Autodesk Inventor part; units mm, degrees
(part 4 of 7)
  arc A284 (154.8425, 86.3766) -> (155.0844, 86.0651) centre (160.0222, 90.1488) ccw projected
  arc A285 (154.6673, 86.6328) -> (154.8425, 86.3766) centre (159.1041, 89.4801) ccw projected
  arc A286 (154.3066, 86.5156) -> (154.6673, 86.6328) centre (148.5, 105) ccw projected
  arc A287 (154.3154, 86.2053) -> (154.3066, 86.5156) centre (149.0434, 86.2112) ccw projected
  arc A288 (154.3028, 85.8111) -> (154.3154, 86.2053) centre (147.9076, 86.2125) ccw projected
  arc A289 (154.2565, 85.3248) -> (154.3028, 85.8111) centre (146.7304, 86.2864) ccw projected
  arc A290 (153.872, 85.2164) -> (154.2565, 85.3248) centre (148.5, 105) ccw projected
  arc A291 (153.5785, 85.6068) -> (153.872, 85.2164) centre (159.7867, 89.9687) ccw projected
  arc A292 (153.3618, 85.9364) -> (153.5785, 85.6068) centre (158.8215, 89.2905) ccw projected
  arc A293 (153.2072, 86.2055) -> (153.3618, 85.9364) centre (157.8537, 88.696) ccw projected
  arc A294 (152.8384, 86.117) -> (153.2072, 86.2055) centre (148.5, 105) ccw projected
  arc A295 (152.8228, 85.807) -> (152.8384, 86.117) centre (147.5676, 86.2265) ccw projected
  arc A296 (152.7793, 85.415) -> (152.8228, 85.807) centre (146.4354, 86.3169) ccw projected
  arc A297 (152.6951, 84.9338) -> (152.7793, 85.415) centre (145.2676, 86.483) ccw projected
  arc A298 (152.3033, 84.8559) -> (152.6951, 84.9338) centre (148.5, 105) ccw projected
  arc A299 (152.0413, 85.2682) -> (152.3033, 84.8559) centre (158.5726, 89.1295) ccw projected
  arc A300 (151.8511, 85.6137) -> (152.0413, 85.2682) centre (157.5571, 88.5292) ccw projected
  arc A301 (151.7181, 85.8941) -> (151.8511, 85.6137) centre (156.5457, 88.0124) ccw projected
  arc A302 (151.3435, 85.8348) -> (151.7181, 85.8941) centre (148.5, 105) ccw projected
  arc A303 (151.3036, 85.527) -> (151.3435, 85.8348) centre (146.0975, 86.3575) ccw projected
  arc A304 (151.2295, 85.1396) -> (151.3036, 85.527) centre (144.9759, 86.5365) ccw projected
  arc A305 (151.1078, 84.6665) -> (151.2295, 85.1396) centre (143.8247, 86.7936) ccw projected
  arc A306 (150.7111, 84.6196) -> (151.1078, 84.6665) centre (148.5, 105) ccw projected
  arc A307 (150.4822, 85.0511) -> (150.7111, 84.6196) centre (157.2963, 88.3881) ccw projected
  arc A308 (150.3197, 85.4105) -> (150.4822, 85.0511) centre (156.2369, 87.8693) ccw projected
  arc A309 (150.2091, 85.7005) -> (150.3197, 85.4105) centre (155.1881, 87.4335) ccw projected
  arc A310 (149.831, 85.6708) -> (150.2091, 85.7005) centre (148.5, 105) ccw projected
  arc A311 (149.7671, 85.367) -> (149.831, 85.6708) centre (144.6423, 86.6035) ccw projected
  arc A312 (149.6629, 84.9867) -> (149.7671, 85.367) centre (143.5382, 86.8699) ccw projected
  arc A313 (149.5044, 84.5246) -> (149.6629, 84.9867) centre (142.4106, 87.2166) ccw projected
  arc A314 (149.1052, 84.5089) -> (149.5044, 84.5246) centre (148.5, 105) ccw projected
  arc A315 (148.9109, 84.9571) -> (149.1052, 84.5089) centre (155.9658, 87.7492) ccw projected
  arc A316 (148.7771, 85.3281) -> (148.9109, 84.9571) centre (154.869, 87.3151) ccw projected
  arc A317 (148.6896, 85.6259) -> (148.7771, 85.3281) centre (153.7892, 86.9629) ccw projected
  arc A318 (148.3104, 85.6259) -> (148.6896, 85.6259) centre (148.5, 105) ccw projected
  arc A319 (148.2229, 85.3281) -> (148.3104, 85.6259) centre (143.2108, 86.9629) ccw projected
  arc A320 (148.0891, 84.9571) -> (148.2229, 85.3281) centre (142.131, 87.3151) ccw projected
  arc A321 (147.8948, 84.5089) -> (148.0891, 84.9571) centre (141.0342, 87.7492) ccw projected
  arc A322 (147.4956, 84.5246) -> (147.8948, 84.5089) centre (148.5, 105) ccw projected
  arc A323 (147.3371, 84.9867) -> (147.4956, 84.5246) centre (154.5894, 87.2166) ccw projected
  arc A324 (147.2329, 85.367) -> (147.3371, 84.9867) centre (153.4618, 86.8699) ccw projected
  arc A325 (147.169, 85.6708) -> (147.2329, 85.367) centre (152.3577, 86.6035) ccw projected
  arc A326 (146.7909, 85.7005) -> (147.169, 85.6708) centre (148.5, 105) ccw projected
  arc A327 (146.6803, 85.4105) -> (146.7909, 85.7005) centre (141.8119, 87.4335) ccw projected
  arc A328 (146.5178, 85.0511) -> (146.6803, 85.4105) centre (140.7631, 87.8693) ccw projected
  arc A329 (146.2889, 84.6196) -> (146.5178, 85.0511) centre (139.7037, 88.3881) ccw projected
  arc A330 (145.8922, 84.6665) -> (146.2889, 84.6196) centre (148.5, 105) ccw projected
  arc A331 (145.7705, 85.1396) -> (145.8922, 84.6665) centre (153.1753, 86.7936) ccw projected
  arc A332 (145.6964, 85.527) -> (145.7705, 85.1396) centre (152.0241, 86.5365) ccw projected
  arc A333 (145.6565, 85.8348) -> (145.6964, 85.527) centre (150.9025, 86.3575) ccw projected
  arc A334 (145.2819, 85.8941) -> (145.6565, 85.8348) centre (148.5, 105) ccw projected
  arc A335 (145.1489, 85.6137) -> (145.2819, 85.8941) centre (140.4543, 88.0124) ccw projected
  arc A336 (144.9587, 85.2682) -> (145.1489, 85.6137) centre (139.4429, 88.5292) ccw projected
  arc A337 (144.6967, 84.8559) -> (144.9587, 85.2682) centre (138.4274, 89.1295) ccw projected
  arc A338 (144.3049, 84.9338) -> (144.6967, 84.8559) centre (148.5, 105) ccw projected
  arc A339 (144.2207, 85.415) -> (144.3049, 84.9338) centre (151.7324, 86.483) ccw projected
  arc A340 (144.1772, 85.807) -> (144.2207, 85.415) centre (150.5646, 86.3169) ccw projected
  arc A341 (144.1616, 86.117) -> (144.1772, 85.807) centre (149.4324, 86.2265) ccw projected
  arc A342 (143.7928, 86.2055) -> (144.1616, 86.117) centre (148.5, 105) ccw projected
  arc A343 (143.6382, 85.9364) -> (143.7928, 86.2055) centre (139.1463, 88.696) ccw projected
  arc A344 (143.4215, 85.6068) -> (143.6382, 85.9364) centre (138.1785, 89.2905) ccw projected
  arc A345 (143.128, 85.2164) -> (143.4215, 85.6068) centre (137.2133, 89.9687) ccw projected
  arc A346 (142.7435, 85.3248) -> (143.128, 85.2164) centre (148.5, 105) ccw projected
  arc A347 (142.6972, 85.8111) -> (142.7435, 85.3248) centre (150.2696, 86.2864) ccw projected
  arc A348 (142.6846, 86.2053) -> (142.6972, 85.8111) centre (149.0924, 86.2125) ccw projected
  arc A349 (142.6934, 86.5156) -> (142.6846, 86.2053) centre (147.9566, 86.2112) ccw projected
  arc A350 (142.3327, 86.6328) -> (142.6934, 86.5156) centre (148.5, 105) ccw projected
  arc A351 (142.1575, 86.3766) -> (142.3327, 86.6328) centre (137.8959, 89.4801) ccw projected
  arc A352 (141.9156, 86.0651) -> (142.1575, 86.3766) centre (136.9778, 90.1488) ccw projected
  arc A353 (141.5923, 85.6989) -> (141.9156, 86.0651) centre (136.0688, 90.9006) ccw projected
  arc A354 (141.2175, 85.8371) -> (141.5923, 85.6989) centre (148.5, 105) ccw projected
  arc A355 (141.2096, 86.3255) -> (141.2175, 85.8371) centre (148.7959, 86.2053) ccw projected
  arc A356 (141.228, 86.7195) -> (141.2096, 86.3255) centre (147.6165, 86.224) ccw projected
  arc A357 (141.2611, 87.0281) -> (141.228, 86.7195) centre (146.4841, 86.3118) ccw projected
  arc A358 (140.9107, 87.1733) -> (141.2611, 87.0281) centre (148.5, 105) ccw projected
  arc A359 (140.7158, 86.9316) -> (140.9107, 87.1733) centre (136.7109, 90.36) ccw projected
  arc A360 (140.4503, 86.64) -> (140.7158, 86.9316) centre (135.8481, 91.0986) ccw projected
  arc A361 (140.0993, 86.3003) -> (140.4503, 86.64) centre (135.0009, 91.9194) ccw projected
  arc A362 (139.7365, 86.4676) -> (140.0993, 86.3003) centre (148.5, 105) ccw projected
  arc A363 (139.7669, 86.9551) -> (139.7365, 86.4676) centre (147.3204, 86.24) ccw projected
  arc A364 (139.8161, 87.3464) -> (139.7669, 86.9551) centre (146.1461, 86.3512) ccw projected
  arc A365 (139.8733, 87.6515) -> (139.8161, 87.3464) centre (145.024, 86.5276) ccw projected
  arc A366 (139.5354, 87.8237) -> (139.8733, 87.6515) centre (148.5, 105) ccw projected
  arc A367 (139.3222, 87.5981) -> (139.5354, 87.8237) centre (135.5986, 91.3301) ccw projected
  arc A368 (139.0346, 87.3282) -> (139.3222, 87.5981) centre (134.7964, 92.1341) ccw projected
  arc A369 (138.658, 87.0171) -> (139.0346, 87.3282) centre (134.0162, 93.0188) ccw projected
  arc A370 (138.3095, 87.2123) -> (138.658, 87.0171) centre (148.5, 105) ccw projected
  arc A371 (138.378, 87.6959) -> (138.3095, 87.2123) centre (145.8522, 86.3904) ccw projected
  arc A372 (138.4578, 88.0822) -> (138.378, 87.6959) centre (144.6901, 86.5933) ccw projected
  arc A373 (138.5388, 88.3818) -> (138.4578, 88.0822) centre (143.5854, 86.8572) ccw projected
  arc A374 (138.2154, 88.58) -> (138.5388, 88.3818) centre (148.5, 105) ccw projected
  arc A375 (137.9852, 88.3718) -> (138.2154, 88.58) centre (134.5659, 92.3844) ccw projected
  arc A376 (137.6773, 88.1253) -> (137.9852, 88.3718) centre (133.8292, 93.2489) ccw projected
  arc A377 (137.2774, 87.8447) -> (137.6773, 88.1253) centre (133.1208, 94.1922) ccw projected
  arc A378 (136.9453, 88.0666) -> (137.2774, 87.8447) centre (148.5, 105) ccw projected
  arc A379 (137.0515, 88.5434) -> (136.9453, 88.0666) centre (144.4002, 86.6555) ccw projected
  arc A380 (137.1614, 88.9222) -> (137.0515, 88.5434) centre (143.2577, 86.949) ccw projected
  arc A381 (137.2656, 89.2146) -> (137.1614, 88.9222) centre (142.1771, 87.2988) ccw projected
  arc A382 (136.9588, 89.4375) -> (137.2656, 89.2146) centre (148.5, 105) ccw projected
  arc A383 (136.7129, 89.248) -> (136.9588, 89.4375) centre (133.619, 93.5166) ccw projected
  arc A384 (136.3866, 89.0265) -> (136.7129, 89.248) centre (132.9524, 94.4362) ccw projected
  arc A385 (135.966, 88.7781) -> (136.3866, 89.0265) centre (132.3202, 95.4321) ccw projected
  arc A386 (135.6523, 89.0254) -> (135.966, 88.7781) centre (148.5, 105) ccw projected
  arc A387 (135.7957, 89.4924) -> (135.6523, 89.0254) centre (142.9736, 87.0337) ccw projected
  arc A388 (135.9349, 89.8614) -> (135.7957, 89.4924) centre (141.8576, 87.4159) ccw projected
  arc A389 (136.0617, 90.1447) -> (135.9349, 89.8614) centre (140.8078, 87.8494) ccw projected
  arc A390 (135.7734, 90.391) -> (136.0617, 90.1447) centre (148.5, 105) ccw projected
  arc A391 (135.5134, 90.2214) -> (135.7734, 90.391) centre (132.7639, 94.7195) ccw projected
  arc A392 (135.1707, 90.0261) -> (135.5134, 90.2214) centre (132.1715, 95.6886) ccw projected
  arc A393 (134.7319, 89.8115) -> (135.1707, 90.0261) centre (131.6194, 96.7311) ccw projected
  arc A394 (134.4386, 90.0827) -> (134.7319, 89.8115) centre (148.5, 105) ccw projected
  arc A395 (134.6181, 90.537) -> (134.4386, 90.0827) centre (141.581, 87.5227) ccw projected
  arc A396 (134.7859, 90.8939) -> (134.6181, 90.537) centre (140.4985, 87.9913) ccw projected
  arc A397 (134.9345, 91.1664) -> (134.7859, 90.8939) centre (139.4859, 88.5058) ccw projected
  arc A398 (134.6664, 91.4345) -> (134.9345, 91.1664) centre (148.5, 105) ccw projected
  arc A399 (134.3939, 91.2859) -> (134.6664, 91.4345) centre (132.0058, 95.9859) ccw projected
  arc A400 (134.037, 91.1181) -> (134.3939, 91.2859) centre (131.4913, 96.9985) ccw projected
  arc A401 (133.5827, 90.9386) -> (134.037, 91.1181) centre (131.0227, 98.081) ccw projected
  arc A402 (133.3115, 91.2319) -> (133.5827, 90.9386) centre (148.5, 105) ccw projected
  arc A403 (133.5261, 91.6707) -> (133.3115, 91.2319) centre (140.2311, 88.1194) ccw projected
  arc A404 (133.7214, 92.0134) -> (133.5261, 91.6707) centre (139.1886, 88.6715) ccw projected
  arc A405 (133.891, 92.2734) -> (133.7214, 92.0134) centre (138.2195, 89.2639) ccw projected
  arc A406 (133.6447, 92.5617) -> (133.891, 92.2734) centre (148.5, 105) ccw projected
  arc A407 (133.3614, 92.4349) -> (133.6447, 92.5617) centre (131.3494, 97.3078) ccw projected
  arc A408 (132.9924, 92.2957) -> (133.3614, 92.4349) centre (130.9159, 98.3576) ccw projected
  arc A409 (132.5254, 92.1523) -> (132.9924, 92.2957) centre (130.5337, 99.4736) ccw projected
  arc A410 (132.2781, 92.466) -> (132.5254, 92.1523) centre (148.5, 105) ccw projected
  arc A411 (132.5265, 92.8866) -> (132.2781, 92.466) centre (138.9321, 88.8202) ccw projected
  arc A412 (132.748, 93.2129) -> (132.5265, 92.8866) centre (137.9362, 89.4524) ccw projected
  arc A413 (132.9375, 93.4588) -> (132.748, 93.2129) centre (137.0166, 90.119) ccw projected
  arc A414 (132.7146, 93.7656) -> (132.9375, 93.4588) centre (148.5, 105) ccw projected
  arc A415 (132.4222, 93.6614) -> (132.7146, 93.7656) centre (130.7988, 98.6771) ccw projected
  arc A416 (132.0434, 93.5515) -> (132.4222, 93.6614) centre (130.449, 99.7577) ccw projected
  arc A417 (131.5666, 93.4453) -> (132.0434, 93.5515) centre (130.1555, 100.9002) ccw projected
  arc A418 (131.3447, 93.7774) -> (131.5666, 93.4453) centre (148.5, 105) ccw projected
  arc A419 (131.6253, 94.1773) -> (131.3447, 93.7774) centre (137.6922, 89.6208) ccw projected
  arc A420 (131.8718, 94.4852) -> (131.6253, 94.1773) centre (136.7489, 90.3292) ccw projected
  arc A421 (132.08, 94.7154) -> (131.8718, 94.4852) centre (135.8844, 91.0659) ccw projected
  arc A422 (131.8818, 95.0388) -> (132.08, 94.7154) centre (148.5, 105) ccw projected
  arc A423 (131.5822, 94.9578) -> (131.8818, 95.0388) centre (130.3572, 100.0854) ccw projected
  arc A424 (131.1959, 94.878) -> (131.5822, 94.9578) centre (130.0933, 101.1901) ccw projected
  arc A425 (130.7123, 94.8095) -> (131.1959, 94.878) centre (129.8904, 102.3522) ccw projected
  arc A426 (130.5171, 95.158) -> (130.7123, 94.8095) centre (148.5, 105) ccw projected
  arc A427 (130.8282, 95.5346) -> (130.5171, 95.158) centre (136.5188, 90.5162) ccw projected
  arc A428 (131.0981, 95.8222) -> (130.8282, 95.5346) centre (135.6341, 91.2964) ccw projected
  arc A429 (131.3237, 96.0354) -> (131.0981, 95.8222) centre (134.8301, 92.0986) ccw projected
  arc A430 (131.1515, 96.3733) -> (131.3237, 96.0354) centre (148.5, 105) ccw projected
  arc A431 (130.8464, 96.3161) -> (131.1515, 96.3733) centre (130.0276, 101.524) ccw projected
  arc A432 (130.4551, 96.2669) -> (130.8464, 96.3161) centre (129.8512, 102.6461) ccw projected
  arc A433 (129.9676, 96.2365) -> (130.4551, 96.2669) centre (129.74, 103.8204) ccw projected
  arc A434 (129.8003, 96.5993) -> (129.9676, 96.2365) centre (148.5, 105) ccw projected
  arc A435 (130.14, 96.9503) -> (129.8003, 96.5993) centre (135.4194, 91.5009) ccw projected
  arc A436 (130.4316, 97.2158) -> (130.14, 96.9503) centre (134.5986, 92.3481) ccw projected
  arc A437 (130.6733, 97.4107) -> (130.4316, 97.2158) centre (133.86, 93.2109) ccw projected
  arc A438 (130.5281, 97.7611) -> (130.6733, 97.4107) centre (148.5, 105) ccw projected
  arc A439 (130.2195, 97.728) -> (130.5281, 97.7611) centre (129.8118, 102.9841) ccw projected
  arc A440 (129.8255, 97.7096) -> (130.2195, 97.728) centre (129.724, 104.1165) ccw projected
  arc A441 (129.3371, 97.7175) -> (129.8255, 97.7096) centre (129.7053, 105.2959) ccw projected
  arc A442 (129.1989, 98.0923) -> (129.3371, 97.7175) centre (148.5, 105) ccw projected
  arc A443 (129.5651, 98.4156) -> (129.1989, 98.0923) centre (134.4006, 92.5688) ccw projected
  arc A444 (129.8766, 98.6575) -> (129.5651, 98.4156) centre (133.6488, 93.4778) ccw projected
  arc A445 (130.1328, 98.8327) -> (129.8766, 98.6575) centre (132.9801, 94.3959) ccw projected
  arc A446 (130.0156, 99.1934) -> (130.1328, 98.8327) centre (148.5, 105) ccw projected
  arc A447 (129.7053, 99.1846) -> (130.0156, 99.1934) centre (129.7112, 104.4566) ccw projected
  arc A448 (129.3111, 99.1972) -> (129.7053, 99.1846) centre (129.7125, 105.5924) ccw projected
  arc A449 (128.8248, 99.2435) -> (129.3111, 99.1972) centre (129.7864, 106.7696) ccw projected
  arc A450 (128.7164, 99.628) -> (128.8248, 99.2435) centre (148.5, 105) ccw projected
  arc A451 (129.1068, 99.9215) -> (128.7164, 99.628) centre (133.4687, 93.7133) ccw projected
  arc A452 (129.4364, 100.1382) -> (129.1068, 99.9215) centre (132.7905, 94.6785) ccw projected
  arc A453 (129.7055, 100.2928) -> (129.4364, 100.1382) centre (132.196, 95.6463) ccw projected
  arc A454 (129.617, 100.6616) -> (129.7055, 100.2928) centre (148.5, 105) ccw projected
  arc A455 (129.307, 100.6772) -> (129.617, 100.6616) centre (129.7265, 105.9324) ccw projected
  arc A456 (128.915, 100.7207) -> (129.307, 100.6772) centre (129.8169, 107.0646) ccw projected
  arc A457 (128.4338, 100.8049) -> (128.915, 100.7207) centre (129.983, 108.2324) ccw projected
  arc A458 (128.3559, 101.1967) -> (128.4338, 100.8049) centre (148.5, 105) ccw projected
  arc A459 (128.7682, 101.4587) -> (128.3559, 101.1967) centre (132.6295, 94.9274) ccw projected
  arc A460 (129.1137, 101.6489) -> (128.7682, 101.4587) centre (132.0292, 95.9429) ccw projected
  arc A461 (129.3941, 101.7819) -> (129.1137, 101.6489) centre (131.5124, 96.9543) ccw projected
  arc A462 (129.3348, 102.1565) -> (129.3941, 101.7819) centre (148.5, 105) ccw projected
  arc A463 (129.027, 102.1964) -> (129.3348, 102.1565) centre (129.8575, 107.4025) ccw projected
  arc A464 (128.6396, 102.2705) -> (129.027, 102.1964) centre (130.0365, 108.5241) ccw projected
  arc A465 (128.1665, 102.3922) -> (128.6396, 102.2705) centre (130.2936, 109.6753) ccw projected
  arc A466 (128.1196, 102.7889) -> (128.1665, 102.3922) centre (148.5, 105) ccw projected
  arc A467 (128.5511, 103.0178) -> (128.1196, 102.7889) centre (131.8881, 96.2037) ccw projected
  arc A468 (128.9105, 103.1803) -> (128.5511, 103.0178) centre (131.3693, 97.2631) ccw projected
  arc A469 (129.2005, 103.2909) -> (128.9105, 103.1803) centre (130.9335, 98.3119) ccw projected
  arc A470 (129.1708, 103.669) -> (129.2005, 103.2909) centre (148.5, 105) ccw projected
  arc A471 (128.867, 103.7329) -> (129.1708, 103.669) centre (130.1035, 108.8577) ccw projected
  arc A472 (128.4867, 103.8371) -> (128.867, 103.7329) centre (130.3699, 109.9618) ccw projected
  arc A473 (128.0246, 103.9956) -> (128.4867, 103.8371) centre (130.7166, 111.0894) ccw projected
  arc A474 (128.0089, 104.3948) -> (128.0246, 103.9956) centre (148.5, 105) ccw projected
  arc A475 (128.4571, 104.5891) -> (128.0089, 104.3948) centre (131.2492, 97.5342) ccw projected
  arc A476 (128.8281, 104.7229) -> (128.4571, 104.5891) centre (130.8151, 98.631) ccw projected
  arc A477 (129.1259, 104.8104) -> (128.8281, 104.7229) centre (130.4629, 99.7108) ccw projected
  arc A478 (129.1259, 105.1896) -> (129.1259, 104.8104) centre (148.5, 105) ccw projected
  arc A479 (128.8281, 105.2771) -> (129.1259, 105.1896) centre (130.4629, 110.2892) ccw projected
  arc A480 (128.4571, 105.4109) -> (128.8281, 105.2771) centre (130.8151, 111.369) ccw projected
  arc A481 (128.0089, 105.6052) -> (128.4571, 105.4109) centre (131.2492, 112.4658) ccw projected
  arc A482 (128.0246, 106.0044) -> (128.0089, 105.6052) centre (148.5, 105) ccw projected
  arc A483 (128.4867, 106.1629) -> (128.0246, 106.0044) centre (130.7166, 98.9106) ccw projected
  arc A484 (128.867, 106.2671) -> (128.4867, 106.1629) centre (130.3699, 100.0382) ccw projected
  arc A485 (129.1708, 106.331) -> (128.867, 106.2671) centre (130.1035, 101.1423) ccw projected
  arc A486 (129.2005, 106.7091) -> (129.1708, 106.331) centre (148.5, 105) ccw projected
  arc A487 (128.9105, 106.8197) -> (129.2005, 106.7091) centre (130.9335, 111.6881) ccw projected
  arc A488 (128.5511, 106.9822) -> (128.9105, 106.8197) centre (131.3693, 112.7369) ccw projected
  arc A489 (128.1196, 107.2111) -> (128.5511, 106.9822) centre (131.8881, 113.7963) ccw projected
  arc A490 (128.1665, 107.6078) -> (128.1196, 107.2111) centre (148.5, 105) ccw projected
  arc A491 (128.6396, 107.7295) -> (128.1665, 107.6078) centre (130.2936, 100.3247) ccw projected
  arc A492 (129.027, 107.8036) -> (128.6396, 107.7295) centre (130.0365, 101.4759) ccw projected
  arc A493 (129.3348, 107.8435) -> (129.027, 107.8036) centre (129.8575, 102.5975) ccw projected
  arc A494 (129.3941, 108.2181) -> (129.3348, 107.8435) centre (148.5, 105) ccw projected
  arc A495 (129.1137, 108.3511) -> (129.3941, 108.2181) centre (131.5124, 113.0457) ccw projected
  arc A496 (128.7682, 108.5413) -> (129.1137, 108.3511) centre (132.0292, 114.0571) ccw projected
  arc A497 (128.3559, 108.8033) -> (128.7682, 108.5413) centre (132.6295, 115.0726) ccw projected
  arc A498 (128.4338, 109.1951) -> (128.3559, 108.8033) centre (148.5, 105) ccw projected
  arc A499 (128.915, 109.2793) -> (128.4338, 109.1951) centre (129.983, 101.7676) ccw projected
  arc A500 (129.307, 109.3228) -> (128.915, 109.2793) centre (129.8169, 102.9354) ccw projected
  arc A501 (129.617, 109.3384) -> (129.307, 109.3228) centre (129.7265, 104.0676) ccw projected
  arc A502 (129.7055, 109.7072) -> (129.617, 109.3384) centre (148.5, 105) ccw projected
  arc A503 (129.4364, 109.8618) -> (129.7055, 109.7072) centre (132.196, 114.3537) ccw projected
  arc A504 (129.1068, 110.0785) -> (129.4364, 109.8618) centre (132.7905, 115.3215) ccw projected
  arc A505 (128.7164, 110.372) -> (129.1068, 110.0785) centre (133.4687, 116.2867) ccw projected
  arc A506 (128.8248, 110.7565) -> (128.7164, 110.372) centre (148.5, 105) ccw projected
  arc A507 (129.3111, 110.8028) -> (128.8248, 110.7565) centre (129.7864, 103.2304) ccw projected
  arc A508 (129.7053, 110.8154) -> (129.3111, 110.8028) centre (129.7125, 104.4076) ccw projected
  arc A509 (130.0156, 110.8066) -> (129.7053, 110.8154) centre (129.7112, 105.5434) ccw projected
  arc A510 (130.1328, 111.1673) -> (130.0156, 110.8066) centre (148.5, 105) ccw projected
  arc A511 (129.8766, 111.3425) -> (130.1328, 111.1673) centre (132.9801, 115.6041) ccw projected
  arc A512 (129.5651, 111.5844) -> (129.8766, 111.3425) centre (133.6488, 116.5222) ccw projected
  arc A513 (129.1989, 111.9077) -> (129.5651, 111.5844) centre (134.4006, 117.4312) ccw projected
  arc A514 (129.3371, 112.2825) -> (129.1989, 111.9077) centre (148.5, 105) ccw projected
  arc A515 (129.8255, 112.2904) -> (129.3371, 112.2825) centre (129.7053, 104.7041) ccw projected
  arc A516 (130.2195, 112.272) -> (129.8255, 112.2904) centre (129.724, 105.8835) ccw projected
  arc A517 (130.5281, 112.2389) -> (130.2195, 112.272) centre (129.8118, 107.0159) ccw projected
  arc A518 (130.6733, 112.5893) -> (130.5281, 112.2389) centre (148.5, 105) ccw projected
  arc A519 (130.4316, 112.7842) -> (130.6733, 112.5893) centre (133.86, 116.7891) ccw projected
  arc A520 (130.14, 113.0497) -> (130.4316, 112.7842) centre (134.5986, 117.6519) ccw projected
  arc A521 (129.8003, 113.4007) -> (130.14, 113.0497) centre (135.4194, 118.4991) ccw projected
  arc A522 (129.9676, 113.7635) -> (129.8003, 113.4007) centre (148.5, 105) ccw projected
  arc A523 (130.4551, 113.7331) -> (129.9676, 113.7635) centre (129.74, 106.1796) ccw projected
  arc A524 (130.8464, 113.6839) -> (130.4551, 113.7331) centre (129.8512, 107.3539) ccw projected
  arc A525 (131.1515, 113.6267) -> (130.8464, 113.6839) centre (130.0276, 108.476) ccw projected
  arc A526 (131.3237, 113.9646) -> (131.1515, 113.6267) centre (148.5, 105) ccw projected
  arc A527 (131.0981, 114.1778) -> (131.3237, 113.9646) centre (134.8301, 117.9014) ccw projected
  arc A528 (130.8282, 114.4654) -> (131.0981, 114.1778) centre (135.6341, 118.7036) ccw projected
  arc A529 (130.5171, 114.842) -> (130.8282, 114.4654) centre (136.5188, 119.4838) ccw projected
  arc A530 (130.7123, 115.1905) -> (130.5171, 114.842) centre (148.5, 105) ccw projected
  arc A531 (131.1959, 115.122) -> (130.7123, 115.1905) centre (129.8904, 107.6478) ccw projected
  arc A532 (131.5822, 115.0422) -> (131.1959, 115.122) centre (130.0933, 108.8099) ccw projected
  arc A533 (131.8818, 114.9612) -> (131.5822, 115.0422) centre (130.3572, 109.9146) ccw projected
  arc A534 (132.08, 115.2846) -> (131.8818, 114.9612) centre (148.5, 105) ccw projected
  arc A535 (131.8718, 115.5148) -> (132.08, 115.2846) centre (135.8844, 118.9341) ccw projected
  arc A536 (131.6253, 115.8227) -> (131.8718, 115.5148) centre (136.7489, 119.6708) ccw projected
  arc A537 (131.3447, 116.2226) -> (131.6253, 115.8227) centre (137.6922, 120.3792) ccw projected
  arc A538 (131.5666, 116.5547) -> (131.3447, 116.2226) centre (148.5, 105) ccw projected
  arc A539 (132.0434, 116.4485) -> (131.5666, 116.5547) centre (130.1555, 109.0998) ccw projected
  arc A540 (132.4222, 116.3386) -> (132.0434, 116.4485) centre (130.449, 110.2423) ccw projected
  arc A541 (132.7146, 116.2344) -> (132.4222, 116.3386) centre (130.7988, 111.3229) ccw projected
  arc A542 (132.9375, 116.5412) -> (132.7146, 116.2344) centre (148.5, 105) ccw projected
  arc A543 (132.748, 116.7871) -> (132.9375, 116.5412) centre (137.0166, 119.881) ccw projected
  arc A544 (132.5265, 117.1134) -> (132.748, 116.7871) centre (137.9362, 120.5476) ccw projected
  arc A545 (132.2781, 117.534) -> (132.5265, 117.1134) centre (138.9321, 121.1798) ccw projected
  arc A546 (132.5254, 117.8477) -> (132.2781, 117.534) centre (148.5, 105) ccw projected
  arc A547 (132.9924, 117.7043) -> (132.5254, 117.8477) centre (130.5337, 110.5264) ccw projected
  arc A548 (133.3614, 117.5651) -> (132.9924, 117.7043) centre (130.9159, 111.6424) ccw projected
  arc A549 (133.6447, 117.4383) -> (133.3614, 117.5651) centre (131.3494, 112.6922) ccw projected
  arc A550 (133.891, 117.7266) -> (133.6447, 117.4383) centre (148.5, 105) ccw projected
  arc A551 (133.7214, 117.9866) -> (133.891, 117.7266) centre (138.2195, 120.7361) ccw projected
  arc A552 (133.5261, 118.3293) -> (133.7214, 117.9866) centre (139.1886, 121.3285) ccw projected
  arc A553 (133.3115, 118.7681) -> (133.5261, 118.3293) centre (140.2311, 121.8806) ccw projected
  arc A554 (133.5827, 119.0614) -> (133.3115, 118.7681) centre (148.5, 105) ccw projected
  arc A555 (134.037, 118.8819) -> (133.5827, 119.0614) centre (131.0227, 111.919) ccw projected
  arc A556 (134.3939, 118.7141) -> (134.037, 118.8819) centre (131.4913, 113.0015) ccw projected
  arc A557 (134.6664, 118.5655) -> (134.3939, 118.7141) centre (132.0058, 114.0141) ccw projected
  arc A558 (134.9345, 118.8336) -> (134.6664, 118.5655) centre (148.5, 105) ccw projected
  arc A559 (134.7859, 119.1061) -> (134.9345, 118.8336) centre (139.4859, 121.4942) ccw projected
  arc A560 (134.6181, 119.463) -> (134.7859, 119.1061) centre (140.4985, 122.0087) ccw projected
  arc A561 (134.4386, 119.9173) -> (134.6181, 119.463) centre (141.581, 122.4773) ccw projected
  arc A562 (134.7319, 120.1885) -> (134.4386, 119.9173) centre (148.5, 105) ccw projected
  arc A563 (135.1707, 119.9739) -> (134.7319, 120.1885) centre (131.6194, 113.2689) ccw projected
  arc A564 (135.5134, 119.7786) -> (135.1707, 119.9739) centre (132.1715, 114.3114) ccw projected
  arc A565 (135.7734, 119.609) -> (135.5134, 119.7786) centre (132.7639, 115.2805) ccw projected
  arc A566 (136.0617, 119.8553) -> (135.7734, 119.609) centre (148.5, 105) ccw projected
  arc A567 (135.9349, 120.1386) -> (136.0617, 119.8553) centre (140.8078, 122.1506) ccw projected
  arc A568 (135.7957, 120.5076) -> (135.9349, 120.1386) centre (141.8576, 122.5841) ccw projected
  arc A569 (135.6523, 120.9746) -> (135.7957, 120.5076) centre (142.9736, 122.9663) ccw projected
  arc A570 (135.966, 121.2219) -> (135.6523, 120.9746) centre (148.5, 105) ccw projected
  arc A571 (136.3866, 120.9735) -> (135.966, 121.2219) centre (132.3202, 114.5679) ccw projected
  arc A572 (136.7129, 120.752) -> (136.3866, 120.9735) centre (132.9524, 115.5638) ccw projected
  arc A573 (136.9588, 120.5625) -> (136.7129, 120.752) centre (133.619, 116.4834) ccw projected
  arc A574 (137.2656, 120.7854) -> (136.9588, 120.5625) centre (148.5, 105) ccw projected
  arc A575 (137.1614, 121.0778) -> (137.2656, 120.7854) centre (142.1771, 122.7012) ccw projected
  arc A576 (137.0515, 121.4566) -> (137.1614, 121.0778) centre (143.2577, 123.051) ccw projected
  arc A577 (136.9453, 121.9334) -> (137.0515, 121.4566) centre (144.4002, 123.3445) ccw projected
  arc A578 (137.2774, 122.1553) -> (136.9453, 121.9334) centre (148.5, 105) ccw projected
  arc A579 (137.6773, 121.8747) -> (137.2774, 122.1553) centre (133.1208, 115.8078) ccw projected
  arc A580 (137.9852, 121.6282) -> (137.6773, 121.8747) centre (133.8292, 116.7511) ccw projected
  arc A581 (138.2154, 121.42) -> (137.9852, 121.6282) centre (134.5659, 117.6156) ccw projected
  arc A582 (138.5388, 121.6182) -> (138.2154, 121.42) centre (148.5, 105) ccw projected
  arc A583 (138.4578, 121.9178) -> (138.5388, 121.6182) centre (143.5854, 123.1428) ccw projected
  arc A584 (138.378, 122.3041) -> (138.4578, 121.9178) centre (144.6901, 123.4067) ccw projected
  arc A585 (138.3095, 122.7877) -> (138.378, 122.3041) centre (145.8522, 123.6096) ccw projected
  arc A586 (138.658, 122.9829) -> (138.3095, 122.7877) centre (148.5, 105) ccw projected
  arc A587 (139.0346, 122.6718) -> (138.658, 122.9829) centre (134.0162, 116.9812) ccw projected
  arc A588 (139.3222, 122.4019) -> (139.0346, 122.6718) centre (134.7964, 117.8659) ccw projected
  arc A589 (139.5354, 122.1763) -> (139.3222, 122.4019) centre (135.5986, 118.6699) ccw projected
  arc A590 (139.8733, 122.3485) -> (139.5354, 122.1763) centre (148.5, 105) ccw projected
  arc A591 (139.8161, 122.6536) -> (139.8733, 122.3485) centre (145.024, 123.4724) ccw projected
  arc A592 (139.7669, 123.0449) -> (139.8161, 122.6536) centre (146.1461, 123.6488) ccw projected
  arc A593 (139.7365, 123.5324) -> (139.7669, 123.0449) centre (147.3204, 123.76) ccw projected
  arc A594 (140.0993, 123.6997) -> (139.7365, 123.5324) centre (148.5, 105) ccw projected
  arc A595 (140.4503, 123.36) -> (140.0993, 123.6997) centre (135.0009, 118.0806) ccw projected
  arc A596 (140.7158, 123.0684) -> (140.4503, 123.36) centre (135.8481, 118.9014) ccw projected
  arc A597 (140.9107, 122.8267) -> (140.7158, 123.0684) centre (136.7109, 119.64) ccw projected
  arc A598 (141.2611, 122.9719) -> (140.9107, 122.8267) centre (148.5, 105) ccw projected
  arc A599 (141.228, 123.2805) -> (141.2611, 122.9719) centre (146.4841, 123.6882) ccw projected
  arc A600 (141.2096, 123.6745) -> (141.228, 123.2805) centre (147.6165, 123.776) ccw projected
  arc A601 (141.2175, 124.1629) -> (141.2096, 123.6745) centre (148.7959, 123.7947) ccw projected
  arc A602 (141.5923, 124.3011) -> (141.2175, 124.1629) centre (148.5, 105) ccw projected
  arc A603 (141.9156, 123.9349) -> (141.5923, 124.3011) centre (136.0688, 119.0994) ccw projected
  arc A604 (142.1575, 123.6234) -> (141.9156, 123.9349) centre (136.9778, 119.8512) ccw projected
  arc A605 (142.3327, 123.3672) -> (142.1575, 123.6234) centre (137.8959, 120.5199) ccw projected
  arc A606 (142.6934, 123.4844) -> (142.3327, 123.3672) centre (148.5, 105) ccw projected
  arc A607 (142.6846, 123.7947) -> (142.6934, 123.4844) centre (147.9566, 123.7888) ccw projected
  arc A608 (142.6972, 124.1889) -> (142.6846, 123.7947) centre (149.0924, 123.7875) ccw projected
  arc A609 (142.7435, 124.6752) -> (142.6972, 124.1889) centre (150.2696, 123.7136) ccw projected
  arc A610 (143.128, 124.7836) -> (142.7435, 124.6752) centre (148.5, 105) ccw projected
  arc A611 (143.4215, 124.3932) -> (143.128, 124.7836) centre (137.2133, 120.0313) ccw projected
  arc A612 (143.6382, 124.0636) -> (143.4215, 124.3932) centre (138.1785, 120.7095) ccw projected
  arc A613 (143.7928, 123.7945) -> (143.6382, 124.0636) centre (139.1463, 121.304) ccw projected
  arc A614 (144.1616, 123.883) -> (143.7928, 123.7945) centre (148.5, 105) ccw projected
  arc A615 (144.1772, 124.193) -> (144.1616, 123.883) centre (149.4324, 123.7735) ccw projected
  arc A616 (144.2207, 124.585) -> (144.1772, 124.193) centre (150.5646, 123.6831) ccw projected
  arc A617 (144.3049, 125.0662) -> (144.2207, 124.585) centre (151.7324, 123.517) ccw projected
  arc A618 (144.6967, 125.1441) -> (144.3049, 125.0662) centre (148.5, 105) ccw projected
  arc A619 (144.9587, 124.7318) -> (144.6967, 125.1441) centre (138.4274, 120.8705) ccw projected
  arc A620 (145.1489, 124.3863) -> (144.9587, 124.7318) centre (139.4429, 121.4708) ccw projected
  arc A621 (145.2819, 124.1059) -> (145.1489, 124.3863) centre (140.4543, 121.9876) ccw projected
  arc A622 (145.6565, 124.1652) -> (145.2819, 124.1059) centre (148.5, 105) ccw projected
  arc A623 (145.6964, 124.473) -> (145.6565, 124.1652) centre (150.9025, 123.6425) ccw projected
  arc A624 (145.7705, 124.8604) -> (145.6964, 124.473) centre (152.0241, 123.4635) ccw projected
  arc A625 (145.8922, 125.3335) -> (145.7705, 124.8604) centre (153.1753, 123.2064) ccw projected
  arc A626 (146.2889, 125.3804) -> (145.8922, 125.3335) centre (148.5, 105) ccw projected
  arc A627 (146.5178, 124.9489) -> (146.2889, 125.3804) centre (139.7037, 121.6119) ccw projected
  arc A628 (146.6803, 124.5895) -> (146.5178, 124.9489) centre (140.7631, 122.1307) ccw projected
  arc A629 (146.7909, 124.2995) -> (146.6803, 124.5895) centre (141.8119, 122.5665) ccw projected
  arc A630 (147.169, 124.3292) -> (146.7909, 124.2995) centre (148.5, 105) ccw projected
  arc A631 (147.2329, 124.633) -> (147.169, 124.3292) centre (152.3577, 123.3965) ccw projected
  arc A632 (147.3371, 125.0133) -> (147.2329, 124.633) centre (153.4618, 123.1301) ccw projected
  arc A633 (147.4956, 125.4754) -> (147.3371, 125.0133) centre (154.5894, 122.7834) ccw projected
  arc A634 (147.8948, 125.4911) -> (147.4956, 125.4754) centre (148.5, 105) ccw projected
  arc A635 (148.0891, 125.0429) -> (147.8948, 125.4911) centre (141.0342, 122.2508) ccw projected
  arc A636 (148.2229, 124.6719) -> (148.0891, 125.0429) centre (142.131, 122.6849) ccw projected
  arc A637 (148.3104, 124.3741) -> (148.2229, 124.6719) centre (143.2108, 123.0371) ccw projected
  arc A638 (148.6896, 124.3741) -> (148.3104, 124.3741) centre (148.5, 105) ccw projected
  arc A639 (148.7771, 124.6719) -> (148.6896, 124.3741) centre (153.7892, 123.0371) ccw projected
  circle A640 centre (148.5, 105) radius 6
  circle A641 centre (148.5, 105) radius 18.25
  point P0 (0, 0)
  dimension "d15" = 12
  dimension "d16" = 36.5
  constraints: 2 centre point, 2 coincident
  measures "d15" diameter of A640
  measures "d16" diameter of A641
extrude "押し出し4" cut sketch "スケッチ4" against normal blind 0.75 contours A641
sketch "スケッチ8" plane through (148.5, 105, 3) normal (0, 0, 1) x (1, 0, 0)
  point P0 (-148.5, -105)
sketch "スケッチ9" plane through (148.5, 105, 3) normal (0, 0, 1) x (1, 0, 0)
  arc A0 (0.5552, 3.8616) -> (0.5094, 3.7241) centre (1.0825, 3.6097) ccw
  arc A1 (0.8556, 4.3042) -> (0.5552, 3.8616) centre (2.0633, 3.1615) ccw
  arc A2 (2.0309, 5.0806) -> (0.8556, 4.3042) centre (3.1127, 2.1651) ccw
  arc A3 (-2.338, 3.1232) -> (-2.2731, 2.9935) centre (-1.787, 3.3179) ccw
  arc A4 (-2.4386, 3.6485) -> (-2.338, 3.1232) centre (-0.7765, 3.6944) ccw
  arc A5 (-2.1565, 5.0286) -> (-2.4386, 3.6485) centre (0.6701, 3.732) ccw
  arc A6 (-3.8616, 0.5552) -> (-3.7241, 0.5094) centre (-3.6097, 1.0825) ccw
  arc A7 (-4.3042, 0.8556) -> (-3.8616, 0.5552) centre (-3.1615, 2.0633) ccw
  arc A8 (-5.0806, 2.0309) -> (-4.3042, 0.8556) centre (-2.1651, 3.1127) ccw
  arc A9 (-3.1232, -2.338) -> (-2.9935, -2.2731) centre (-3.3179, -1.787) ccw
  arc A10 (-3.6485, -2.4386) -> (-3.1232, -2.338) centre (-3.6944, -0.7765) ccw
  arc A11 (-5.0286, -2.1565) -> (-3.6485, -2.4386) centre (-3.732, 0.6701) ccw
  arc A12 (-0.5552, -3.8616) -> (-0.5094, -3.7241) centre (-1.0825, -3.6097) ccw
  arc A13 (-0.8556, -4.3042) -> (-0.5552, -3.8616) centre (-2.0633, -3.1615) ccw
  arc A14 (-2.0309, -5.0806) -> (-0.8556, -4.3042) centre (-3.1127, -2.1651) ccw
  arc A15 (2.338, -3.1232) -> (2.2731, -2.9935) centre (1.787, -3.3179) ccw
  arc A16 (2.4386, -3.6485) -> (2.338, -3.1232) centre (0.7765, -3.6944) ccw
  arc A17 (2.1565, -5.0286) -> (2.4386, -3.6485) centre (-0.6701, -3.732) ccw
  arc A18 (3.8616, -0.5552) -> (3.7241, -0.5094) centre (3.6097, -1.0825) ccw
  arc A19 (4.3042, -0.8556) -> (3.8616, -0.5552) centre (3.1615, -2.0633) ccw
  arc A20 (5.0806, -2.0309) -> (4.3042, -0.8556) centre (2.1651, -3.1127) ccw
  arc A21 (3.1232, 2.338) -> (2.9935, 2.2731) centre (3.3179, 1.787) ccw
  arc A22 (3.6485, 2.4386) -> (3.1232, 2.338) centre (3.6944, 0.7765) ccw
  arc A23 (5.0286, 2.1565) -> (3.6485, 2.4386) centre (3.732, -0.6701) ccw
  arc A24 (-0.5094, 3.7241) -> (-0.5552, 3.8616) centre (-1.0825, 3.6097) ccw
  arc A25 (-0.5552, 3.8616) -> (-0.8556, 4.3042) centre (-2.0633, 3.1615) ccw
  arc A26 (-0.8556, 4.3042) -> (-2.0309, 5.0806) centre (-3.1127, 2.1651) ccw
  arc A27 (-2.9935, 2.2731) -> (-3.1232, 2.338) centre (-3.3179, 1.787) ccw
  arc A28 (-3.1232, 2.338) -> (-3.6485, 2.4386) centre (-3.6944, 0.7765) ccw
  arc A29 (-3.6485, 2.4386) -> (-5.0286, 2.1565) centre (-3.732, -0.6701) ccw
  arc A30 (-3.7241, -0.5094) -> (-3.8616, -0.5552) centre (-3.6097, -1.0825) ccw
  arc A31 (-3.8616, -0.5552) -> (-4.3042, -0.8556) centre (-3.1615, -2.0633) ccw
  arc A32 (-4.3042, -0.8556) -> (-5.0806, -2.0309) centre (-2.1651, -3.1127) ccw
  arc A33 (-2.2731, -2.9935) -> (-2.338, -3.1232) centre (-1.787, -3.3179) ccw
  arc A34 (-2.338, -3.1232) -> (-2.4387, -3.6513) centre (-0.7765, -3.6944) ccw
  arc A35 (-2.4387, -3.6513) -> (-2.1565, -5.0286) centre (0.6701, -3.732) ccw
  arc A36 (0.5094, -3.7241) -> (0.5552, -3.8616) centre (1.0825, -3.6097) ccw
  arc A37 (0.5552, -3.8616) -> (0.8556, -4.3042) centre (2.0633, -3.1615) ccw
  arc A38 (0.8556, -4.3042) -> (2.0309, -5.0806) centre (3.1127, -2.1651) ccw
  arc A39 (2.9935, -2.2731) -> (3.1232, -2.338) centre (3.3179, -1.787) ccw
  arc A40 (3.1232, -2.338) -> (3.6485, -2.4386) centre (3.6944, -0.7765) ccw
  arc A41 (3.6485, -2.4386) -> (5.0286, -2.1565) centre (3.732, 0.6701) ccw
  arc A42 (3.7241, 0.5094) -> (3.8616, 0.5552) centre (3.6097, 1.0825) ccw
  arc A43 (3.8616, 0.5552) -> (4.3042, 0.8556) centre (3.1615, 2.0633) ccw
  arc A44 (4.3042, 0.8556) -> (5.0806, 2.0309) centre (2.1651, 3.1127) ccw
  arc A45 (2.2731, 2.9935) -> (2.338, 3.1232) centre (1.787, 3.3179) ccw
  arc A46 (2.338, 3.1232) -> (2.4386, 3.6485) centre (0.7765, 3.6944) ccw
  arc A47 (2.4386, 3.6485) -> (2.1565, 5.0286) centre (-0.6701, 3.732) ccw
  arc A48 (0.4405, 3.22) -> (-0.4405, 3.22) centre (0, 0) ccw
  arc A49 (-1.9654, 2.5884) -> (-2.5884, 1.9654) centre (0, 0) ccw
  arc A50 (-3.22, 0.4405) -> (-3.22, -0.4405) centre (0, 0) ccw
  arc A51 (-2.5884, -1.9654) -> (-1.9654, -2.5884) centre (0, 0) ccw
  arc A52 (-0.4405, -3.22) -> (0.4405, -3.22) centre (0, 0) ccw
  arc A53 (1.9654, -2.5884) -> (2.5884, -1.9654) centre (0, 0) ccw
  arc A54 (3.22, -0.4405) -> (3.22, 0.4405) centre (0, 0) ccw
  arc A55 (2.5884, 1.9654) -> (1.9654, 2.5884) centre (0, 0) ccw
  arc A56 (-2.0309, 5.0806) -> (-2.1565, 5.0286) centre (0, 0) ccw
  arc A57 (-5.0286, 2.1565) -> (-5.0806, 2.0309) centre (0, 0) ccw
  arc A58 (-5.0806, -2.0309) -> (-5.0286, -2.1565) centre (0, 0) ccw
  arc A59 (-2.1565, -5.0286) -> (-2.0309, -5.0806) centre (0, 0) ccw
  arc A60 (2.0309, -5.0806) -> (2.1565, -5.0286) centre (0, 0) ccw
  arc A61 (5.0286, -2.1565) -> (5.0806, -2.0309) centre (0, 0) ccw
  arc A62 (5.0806, 2.0309) -> (5.0286, 2.1565) centre (0, 0) ccw
  arc A63 (2.1565, 5.0286) -> (2.0309, 5.0806) centre (0, 0) ccw
  line L0 (0.4405, 3.22) -> (0.5094, 3.7241)
  line L1 (-1.9654, 2.5884) -> (-2.2731, 2.9935)
  line L2 (-3.22, 0.4405) -> (-3.7241, 0.5094)
  line L3 (-2.5884, -1.9654) -> (-2.9935, -2.2731)
  line L4 (-0.4405, -3.22) -> (-0.5094, -3.7241)
  line L5 (1.9654, -2.5884) -> (2.2731, -2.9935)
  line L6 (3.22, -0.4405) -> (3.7241, -0.5094)
  line L7 (2.5884, 1.9654) -> (2.9935, 2.2731)
  line L8 (-0.4405, 3.22) -> (-0.5094, 3.7241)
  line L9 (-2.5884, 1.9654) -> (-2.9935, 2.2731)
  line L10 (-3.22, -0.4405) -> (-3.7241, -0.5094)
  line L11 (-1.9654, -2.5884) -> (-2.2731, -2.9935)
  line L12 (0.4405, -3.22) -> (0.5094, -3.7241)
  line L13 (2.5884, -1.9654) -> (2.9935, -2.2731)
  line L14 (3.22, 0.4405) -> (3.7241, 0.5094)
  line L15 (1.9654, 2.5884) -> (2.2731, 2.9935)
  line L16 (-7.4715, 0) -> (7.4715, 0)
  line L17 (0, -7.4715) -> (0, 7.4715)
  line L18 (173.9715, 110.4715) -> (243.9715, 110.4715)
  line L19 (173.9715, 102.4715) -> (243.9715, 102.4715)
  line L20 (173.9715, 94.4715) -> (243.9715, 94.4715)
  line L21 (173.9715, 86.4715) -> (243.9715, 86.4715)
  line L22 (173.9715, 78.4715) -> (243.9715, 78.4715)
  line L23 (173.9715, 70.4715) -> (243.9715, 70.4715)
  line L24 (173.9715, 62.4715) -> (243.9715, 62.4715)
  line L25 (173.9715, 54.4715) -> (243.9715, 54.4715)
  line L26 (173.9715, 46.4715) -> (243.9715, 46.4715)
  line L27 (173.9715, 38.4715) -> (243.9715, 38.4715)
  line L28 (173.9715, 30.4715) -> (243.9715, 30.4715)
  line L29 (173.9715, 22.4715) -> (243.9715, 22.4715)
  line L30 (173.9715, 14.4715) -> (243.9715, 14.4715)
  line L31 (173.9715, 110.4715) -> (173.9715, 14.4715)
  line L32 (243.9715, 110.4715) -> (243.9715, 14.4715)
  line L33 (208.9715, 102.4715) -> (208.9715, 14.4715)
  circle A64 centre (0, 0) radius 6 projected
  circle A65 centre (0, 0) radius 18.25 projected
  arc A66 (0.4109, 20.0429) -> (0.2771, 19.6719) centre (6.369, 17.6849) ccw projected
  arc A67 (0.6052, 20.4911) -> (0.4109, 20.0429) centre (7.4658, 17.2508) ccw projected
  arc A68 (1.0044, 20.4754) -> (0.6052, 20.4911) centre (0, 0) ccw projected
  arc A69 (1.1629, 20.0133) -> (1.0044, 20.4754) centre (-6.0894, 17.7834) ccw projected
  arc A70 (1.2671, 19.633) -> (1.1629, 20.0133) centre (-4.9618, 18.1301) ccw projected
  arc A71 (1.331, 19.3292) -> (1.2671, 19.633) centre (-3.8577, 18.3965) ccw projected
  arc A72 (1.7091, 19.2995) -> (1.331, 19.3292) centre (0, 0) ccw projected
  arc A73 (1.8197, 19.5895) -> (1.7091, 19.2995) centre (6.6881, 17.5665) ccw projected
  arc A74 (1.9822, 19.9489) -> (1.8197, 19.5895) centre (7.7369, 17.1307) ccw projected
  arc A75 (2.2111, 20.3804) -> (1.9822, 19.9489) centre (8.7963, 16.6119) ccw projected
  arc A76 (2.6078, 20.3335) -> (2.2111, 20.3804) centre (0, 0) ccw projected
  arc A77 (2.7295, 19.8604) -> (2.6078, 20.3335) centre (-4.6753, 18.2064) ccw projected
  arc A78 (2.8036, 19.473) -> (2.7295, 19.8604) centre (-3.5241, 18.4635) ccw projected
  arc A79 (2.8435, 19.1652) -> (2.8036, 19.473) centre (-2.4025, 18.6425) ccw projected
  arc A80 (3.2181, 19.1059) -> (2.8435, 19.1652) centre (0, 0) ccw projected
  arc A81 (3.3511, 19.3863) -> (3.2181, 19.1059) centre (8.0457, 16.9876) ccw projected
  arc A82 (3.5413, 19.7318) -> (3.3511, 19.3863) centre (9.0571, 16.4708) ccw projected
  arc A83 (3.8033, 20.1441) -> (3.5413, 19.7318) centre (10.0726, 15.8705) ccw projected
  arc A84 (4.1951, 20.0662) -> (3.8033, 20.1441) centre (0, 0) ccw projected
  arc A85 (4.2793, 19.585) -> (4.1951, 20.0662) centre (-3.2324, 18.517) ccw projected
  arc A86 (4.3228, 19.193) -> (4.2793, 19.585) centre (-2.0646, 18.6831) ccw projected
  arc A87 (4.3384, 18.883) -> (4.3228, 19.193) centre (-0.9324, 18.7735) ccw projected
  arc A88 (4.7072, 18.7945) -> (4.3384, 18.883) centre (0, 0) ccw projected
  arc A89 (4.8618, 19.0636) -> (4.7072, 18.7945) centre (9.3537, 16.304) ccw projected
  arc A90 (5.0785, 19.3932) -> (4.8618, 19.0636) centre (10.3215, 15.7095) ccw projected
  arc A91 (5.372, 19.7836) -> (5.0785, 19.3932) centre (11.2867, 15.0313) ccw projected
  arc A92 (5.7565, 19.6752) -> (5.372, 19.7836) centre (0, 0) ccw projected
  arc A93 (5.8028, 19.1889) -> (5.7565, 19.6752) centre (-1.7696, 18.7136) ccw projected
  arc A94 (5.8154, 18.7947) -> (5.8028, 19.1889) centre (-0.5924, 18.7875) ccw projected
  arc A95 (5.8066, 18.4844) -> (5.8154, 18.7947) centre (0.5434, 18.7888) ccw projected
  arc A96 (6.1673, 18.3672) -> (5.8066, 18.4844) centre (0, 0) ccw projected
  arc A97 (6.3425, 18.6234) -> (6.1673, 18.3672) centre (10.6041, 15.5199) ccw projected
  arc A98 (6.5844, 18.9349) -> (6.3425, 18.6234) centre (11.5222, 14.8512) ccw projected
  arc A99 (6.9077, 19.3011) -> (6.5844, 18.9349) centre (12.4312, 14.0994) ccw projected
  arc A100 (7.2825, 19.1629) -> (6.9077, 19.3011) centre (0, 0) ccw projected
  arc A101 (7.2904, 18.6745) -> (7.2825, 19.1629) centre (-0.2959, 18.7947) ccw projected
  arc A102 (7.272, 18.2805) -> (7.2904, 18.6745) centre (0.8835, 18.776) ccw projected
  arc A103 (7.2389, 17.9719) -> (7.272, 18.2805) centre (2.0159, 18.6882) ccw projected
  arc A104 (7.5893, 17.8267) -> (7.2389, 17.9719) centre (0, 0) ccw projected
  arc A105 (7.7842, 18.0684) -> (7.5893, 17.8267) centre (11.7891, 14.64) ccw projected
  arc A106 (8.0497, 18.36) -> (7.7842, 18.0684) centre (12.6519, 13.9014) ccw projected
  arc A107 (8.4007, 18.6997) -> (8.0497, 18.36) centre (13.4991, 13.0806) ccw projected
  arc A108 (8.7635, 18.5324) -> (8.4007, 18.6997) centre (0, 0) ccw projected
  arc A109 (8.7331, 18.0449) -> (8.7635, 18.5324) centre (1.1796, 18.76) ccw projected
  arc A110 (8.6839, 17.6536) -> (8.7331, 18.0449) centre (2.3539, 18.6488) ccw projected
  arc A111 (8.6267, 17.3485) -> (8.6839, 17.6536) centre (3.476, 18.4724) ccw projected
  arc A112 (8.9646, 17.1763) -> (8.6267, 17.3485) centre (0, 0) ccw projected
  arc A113 (9.1778, 17.4019) -> (8.9646, 17.1763) centre (12.9014, 13.6699) ccw projected
  arc A114 (9.4654, 17.6718) -> (9.1778, 17.4019) centre (13.7036, 12.8659) ccw projected
  arc A115 (9.842, 17.9829) -> (9.4654, 17.6718) centre (14.4838, 11.9812) ccw projected
  arc A116 (10.1905, 17.7877) -> (9.842, 17.9829) centre (0, 0) ccw projected
  arc A117 (10.122, 17.3041) -> (10.1905, 17.7877) centre (2.6478, 18.6096) ccw projected
  arc A118 (10.0422, 16.9178) -> (10.122, 17.3041) centre (3.8099, 18.4067) ccw projected
  arc A119 (9.9612, 16.6182) -> (10.0422, 16.9178) centre (4.9146, 18.1428) ccw projected
  arc A120 (10.2846, 16.42) -> (9.9612, 16.6182) centre (0, 0) ccw projected
  arc A121 (10.5148, 16.6282) -> (10.2846, 16.42) centre (13.9341, 12.6156) ccw projected
  arc A122 (10.8227, 16.8747) -> (10.5148, 16.6282) centre (14.6708, 11.7511) ccw projected
  arc A123 (11.2226, 17.1553) -> (10.8227, 16.8747) centre (15.3792, 10.8078) ccw projected
  arc A124 (11.5547, 16.9334) -> (11.2226, 17.1553) centre (0, 0) ccw projected
  arc A125 (11.4485, 16.4566) -> (11.5547, 16.9334) centre (4.0998, 18.3445) ccw projected
  arc A126 (11.3386, 16.0778) -> (11.4485, 16.4566) centre (5.2423, 18.051) ccw projected
  arc A127 (11.2344, 15.7854) -> (11.3386, 16.0778) centre (6.3229, 17.7012) ccw projected
  arc A128 (11.5412, 15.5625) -> (11.2344, 15.7854) centre (0, 0) ccw projected
  arc A129 (11.7871, 15.752) -> (11.5412, 15.5625) centre (14.881, 11.4834) ccw projected
  arc A130 (12.1134, 15.9735) -> (11.7871, 15.752) centre (15.5476, 10.5638) ccw projected
  arc A131 (12.534, 16.2219) -> (12.1134, 15.9735) centre (16.1798, 9.5679) ccw projected
  arc A132 (12.8477, 15.9746) -> (12.534, 16.2219) centre (0, 0) ccw projected
  arc A133 (12.7043, 15.5076) -> (12.8477, 15.9746) centre (5.5264, 17.9663) ccw projected
  arc A134 (12.5651, 15.1386) -> (12.7043, 15.5076) centre (6.6424, 17.5841) ccw projected
  arc A135 (12.4383, 14.8553) -> (12.5651, 15.1386) centre (7.6922, 17.1506) ccw projected
  arc A136 (12.7266, 14.609) -> (12.4383, 14.8553) centre (0, 0) ccw projected
  arc A137 (12.9866, 14.7786) -> (12.7266, 14.609) centre (15.7361, 10.2805) ccw projected
  arc A138 (13.3293, 14.9739) -> (12.9866, 14.7786) centre (16.3285, 9.3114) ccw projected
  arc A139 (13.7681, 15.1885) -> (13.3293, 14.9739) centre (16.8806, 8.2689) ccw projected
  arc A140 (14.0614, 14.9173) -> (13.7681, 15.1885) centre (0, 0) ccw projected
  arc A141 (13.8819, 14.463) -> (14.0614, 14.9173) centre (6.919, 17.4773) ccw projected
  arc A142 (13.7141, 14.1061) -> (13.8819, 14.463) centre (8.0015, 17.0087) ccw projected
  arc A143 (13.5655, 13.8336) -> (13.7141, 14.1061) centre (9.0141, 16.4942) ccw projected
  arc A144 (13.8336, 13.5655) -> (13.5655, 13.8336) centre (0, 0) ccw projected
  arc A145 (14.1061, 13.7141) -> (13.8336, 13.5655) centre (16.4942, 9.0141) ccw projected
  arc A146 (14.463, 13.8819) -> (14.1061, 13.7141) centre (17.0087, 8.0015) ccw projected
  arc A147 (14.9173, 14.0614) -> (14.463, 13.8819) centre (17.4773, 6.919) ccw projected
  arc A148 (15.1885, 13.7681) -> (14.9173, 14.0614) centre (0, 0) ccw projected
  arc A149 (14.9739, 13.3293) -> (15.1885, 13.7681) centre (8.2689, 16.8806) ccw projected
  arc A150 (14.7786, 12.9866) -> (14.9739, 13.3293) centre (9.3114, 16.3285) ccw projected
  arc A151 (14.609, 12.7266) -> (14.7786, 12.9866) centre (10.2805, 15.7361) ccw projected
  arc A152 (14.8553, 12.4383) -> (14.609, 12.7266) centre (0, 0) ccw projected
  arc A153 (15.1386, 12.5651) -> (14.8553, 12.4383) centre (17.1506, 7.6922) ccw projected
  arc A154 (15.5076, 12.7043) -> (15.1386, 12.5651) centre (17.5841, 6.6424) ccw projected
  arc A155 (15.9746, 12.8477) -> (15.5076, 12.7043) centre (17.9663, 5.5264) ccw projected
  arc A156 (16.2219, 12.534) -> (15.9746, 12.8477) centre (0, 0) ccw projected
  arc A157 (15.9735, 12.1134) -> (16.2219, 12.534) centre (9.5679, 16.1798) ccw projected
  arc A158 (15.752, 11.7871) -> (15.9735, 12.1134) centre (10.5638, 15.5476) ccw projected
  arc A159 (15.5625, 11.5412) -> (15.752, 11.7871) centre (11.4834, 14.881) ccw projected
  arc A160 (15.7854, 11.2344) -> (15.5625, 11.5412) centre (0, 0) ccw projected
  arc A161 (16.0778, 11.3386) -> (15.7854, 11.2344) centre (17.7012, 6.3229) ccw projected
  arc A162 (16.4566, 11.4485) -> (16.0778, 11.3386) centre (18.051, 5.2423) ccw projected
  arc A163 (16.9334, 11.5547) -> (16.4566, 11.4485) centre (18.3445, 4.0998) ccw projected
  arc A164 (17.1553, 11.2226) -> (16.9334, 11.5547) centre (0, 0) ccw projected
  arc A165 (16.8747, 10.8227) -> (17.1553, 11.2226) centre (10.8078, 15.3792) ccw projected
  arc A166 (16.6282, 10.5148) -> (16.8747, 10.8227) centre (11.7511, 14.6708) ccw projected
  arc A167 (16.42, 10.2846) -> (16.6282, 10.5148) centre (12.6156, 13.9341) ccw projected
  arc A168 (16.6182, 9.9612) -> (16.42, 10.2846) centre (0, 0) ccw projected
  arc A169 (16.9178, 10.0422) -> (16.6182, 9.9612) centre (18.1428, 4.9146) ccw projected
  arc A170 (17.3041, 10.122) -> (16.9178, 10.0422) centre (18.4067, 3.8099) ccw projected
  arc A171 (17.7877, 10.1905) -> (17.3041, 10.122) centre (18.6096, 2.6478) ccw projected
  arc A172 (17.9829, 9.842) -> (17.7877, 10.1905) centre (0, 0) ccw projected
  arc A173 (17.6718, 9.4654) -> (17.9829, 9.842) centre (11.9812, 14.4838) ccw projected
  arc A174 (17.4019, 9.1778) -> (17.6718, 9.4654) centre (12.8659, 13.7036) ccw projected
  arc A175 (17.1763, 8.9646) -> (17.4019, 9.1778) centre (13.6699, 12.9014) ccw projected
  arc A176 (17.3485, 8.6267) -> (17.1763, 8.9646) centre (0, 0) ccw projected
  arc A177 (17.6536, 8.6839) -> (17.3485, 8.6267) centre (18.4724, 3.476) ccw projected
  arc A178 (18.0449, 8.7331) -> (17.6536, 8.6839) centre (18.6488, 2.3539) ccw projected
  arc A179 (18.5324, 8.7635) -> (18.0449, 8.7331) centre (18.76, 1.1796) ccw projected
  arc A180 (18.6997, 8.4007) -> (18.5324, 8.7635) centre (0, 0) ccw projected
  arc A181 (18.36, 8.0497) -> (18.6997, 8.4007) centre (13.0806, 13.4991) ccw projected
  arc A182 (18.0684, 7.7842) -> (18.36, 8.0497) centre (13.9014, 12.6519) ccw projected
  arc A183 (17.8267, 7.5893) -> (18.0684, 7.7842) centre (14.64, 11.7891) ccw projected
  arc A184 (17.9719, 7.2389) -> (17.8267, 7.5893) centre (0, 0) ccw projected
  arc A185 (18.2805, 7.272) -> (17.9719, 7.2389) centre (18.6882, 2.0159) ccw projected
  arc A186 (18.6745, 7.2904) -> (18.2805, 7.272) centre (18.776, 0.8835) ccw projected
  arc A187 (19.1629, 7.2825) -> (18.6745, 7.2904) centre (18.7947, -0.2959) ccw projected
  arc A188 (19.3011, 6.9077) -> (19.1629, 7.2825) centre (0, 0) ccw projected
  arc A189 (18.9349, 6.5844) -> (19.3011, 6.9077) centre (14.0994, 12.4312) ccw projected
  arc A190 (18.6234, 6.3425) -> (18.9349, 6.5844) centre (14.8512, 11.5222) ccw projected
  arc A191 (18.3672, 6.1673) -> (18.6234, 6.3425) centre (15.5199, 10.6041) ccw projected
  arc A192 (18.4844, 5.8066) -> (18.3672, 6.1673) centre (0, 0) ccw projected
  arc A193 (18.7947, 5.8154) -> (18.4844, 5.8066) centre (18.7888, 0.5434) ccw projected
  arc A194 (19.1889, 5.8028) -> (18.7947, 5.8154) centre (18.7875, -0.5924) ccw projected
  arc A195 (19.6752, 5.7565) -> (19.1889, 5.8028) centre (18.7136, -1.7696) ccw projected
  arc A196 (19.7836, 5.372) -> (19.6752, 5.7565) centre (0, 0) ccw projected
  arc A197 (19.3932, 5.0785) -> (19.7836, 5.372) centre (15.0313, 11.2867) ccw projected
  arc A198 (19.0636, 4.8618) -> (19.3932, 5.0785) centre (15.7095, 10.3215) ccw projected
  arc A199 (18.7945, 4.7072) -> (19.0636, 4.8618) centre (16.304, 9.3537) ccw projected
  arc A200 (18.883, 4.3384) -> (18.7945, 4.7072) centre (0, 0) ccw projected
  arc A201 (19.193, 4.3228) -> (18.883, 4.3384) centre (18.7735, -0.9324) ccw projected
  arc A202 (19.585, 4.2793) -> (19.193, 4.3228) centre (18.6831, -2.0646) ccw projected
  arc A203 (20.0662, 4.1951) -> (19.585, 4.2793) centre (18.517, -3.2324) ccw projected
  arc A204 (20.1441, 3.8033) -> (20.0662, 4.1951) centre (0, 0) ccw projected
  arc A205 (19.7318, 3.5413) -> (20.1441, 3.8033) centre (15.8705, 10.0726) ccw projected
  arc A206 (19.3863, 3.3511) -> (19.7318, 3.5413) centre (16.4708, 9.0571) ccw projected
  arc A207 (19.1059, 3.2181) -> (19.3863, 3.3511) centre (16.9876, 8.0457) ccw projected
  arc A208 (19.1652, 2.8435) -> (19.1059, 3.2181) centre (0, 0) ccw projected
  arc A209 (19.473, 2.8036) -> (19.1652, 2.8435) centre (18.6425, -2.4025) ccw projected
  arc A210 (19.8604, 2.7295) -> (19.473, 2.8036) centre (18.4635, -3.5241) ccw projected
  arc A211 (20.3335, 2.6078) -> (19.8604, 2.7295) centre (18.2064, -4.6753) ccw projected
  arc A212 (20.3804, 2.2111) -> (20.3335, 2.6078) centre (0, 0) ccw projected
  arc A213 (19.9489, 1.9822) -> (20.3804, 2.2111) centre (16.6119, 8.7963) ccw projected
  arc A214 (19.5895, 1.8197) -> (19.9489, 1.9822) centre (17.1307, 7.7369) ccw projected
  arc A215 (19.2995, 1.7091) -> (19.5895, 1.8197) centre (17.5665, 6.6881) ccw projected
  arc A216 (19.3292, 1.331) -> (19.2995, 1.7091) centre (0, 0) ccw projected
  arc A217 (19.633, 1.2671) -> (19.3292, 1.331) centre (18.3965, -3.8577) ccw projected
  arc A218 (20.0133, 1.1629) -> (19.633, 1.2671) centre (18.1301, -4.9618) ccw projected
  arc A219 (20.4754, 1.0044) -> (20.0133, 1.1629) centre (17.7834, -6.0894) ccw projected
  arc A220 (20.4911, 0.6052) -> (20.4754, 1.0044) centre (0, 0) ccw projected
  arc A221 (20.0429, 0.4109) -> (20.4911, 0.6052) centre (17.2508, 7.4658) ccw projected
  arc A222 (19.6719, 0.2771) -> (20.0429, 0.4109) centre (17.6849, 6.369) ccw projected
  arc A223 (19.3741, 0.1896) -> (19.6719, 0.2771) centre (18.0371, 5.2892) ccw projected
  arc A224 (19.3741, -0.1896) -> (19.3741, 0.1896) centre (0, 0) ccw projected
  arc A225 (19.6719, -0.2771) -> (19.3741, -0.1896) centre (18.0371, -5.2892) ccw projected
  arc A226 (20.0429, -0.4109) -> (19.6719, -0.2771) centre (17.6849, -6.369) ccw projected
  arc A227 (20.4911, -0.6052) -> (20.0429, -0.4109) centre (17.2508, -7.4658) ccw projected
  arc A228 (20.4754, -1.0044) -> (20.4911, -0.6052) centre (0, 0) ccw projected
  arc A229 (20.0133, -1.1629) -> (20.4754, -1.0044) centre (17.7834, 6.0894) ccw projected
  arc A230 (19.633, -1.2671) -> (20.0133, -1.1629) centre (18.1301, 4.9618) ccw projected
  arc A231 (19.3292, -1.331) -> (19.633, -1.2671) centre (18.3965, 3.8577) ccw projected
  arc A232 (19.2995, -1.7091) -> (19.3292, -1.331) centre (0, 0) ccw projected
  arc A233 (19.5895, -1.8197) -> (19.2995, -1.7091) centre (17.5665, -6.6881) ccw projected